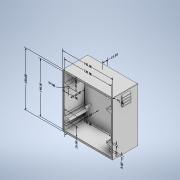
# Autodesk Inventor part: Part_B1
Saved by Autodesk Inventor 2022.6 (Build 266554010, 554A)
## iProperties
Created: 2025-05-15
Part Number: Part_B1
Material: Generic
Document SubType Name: Modeling
Designer: khinm
Density: 1 g/cm^3
Appearance: Default
Author: khinm
Autodesk Inventor part; units mm, degrees
sketch "Sketch1" plane through (0, 0, 0) normal (0, 0, 1) x (1, 0, 0)
  line L0 (-70, 75) -> (70, 75)
  line L1 (70, 75) -> (70, -75)
  line L2 (70, -75) -> (-70, -75)
  line L3 (-70, -75) -> (-70, 75)
  point P0 (0, 0)
  point P1 (-70, 0)
  point P2 (0, 75)
  dimension "d0" = 150
  dimension "d1" = 140
  constraints: 8 end point, 2 midpoint, 2 parallel, 1 horizontal, 1 horizontal alignment, 1 perpendicular, 1 vertical alignment
  measures "d0" distance between parallel lines of L2 L0
  measures "d1" distance between parallel lines of L1 L3
extrude "Extrusion1" add sketch "Sketch1" along normal mid plane 70
sketch "Sketch2" plane through (0, 0, 35) normal (0, 0, 1) x (1, 0, 0)
  line L0 (-65, 70) -> (65, 70)
  line L1 (65, 70) -> (65, -70)
  line L2 (65, -70) -> (-65, -70)
  line L3 (-65, -70) -> (-65, 70)
  point P0 (0, 0)
  point P1 (-65, 0)
  point P2 (0, 70)
  dimension "d4" = 130
  dimension "d5" = 140
  constraints: 8 end point, 2 midpoint, 2 parallel, 1 horizontal, 1 horizontal alignment, 1 perpendicular, 1 vertical alignment
  measures "d4" distance of L0.start L0.end
  measures "d5" distance of L0.end L1.end
extrude "Extrusion2" cut sketch "Sketch2" against normal blind 55
sketch "Sketch4" plane through (0, 0, -20) normal (0, 0, 1) x (1, 0, 0)
  arc A0 (-55, 36) -> (-55, 44) centre (-55, 40) ccw
  arc A1 (-55, -44) -> (-55, -36) centre (-55, -40) ccw
  line L0 (-65, 70) -> (65, 70) projected
  line L1 (65, -70) -> (-65, -70) projected
  line L2 (-65, -70) -> (-65, 70) projected
  line L3 (-55, 44) -> (-65, 44)
  line L4 (-55, 36) -> (-65, 36)
  line L5 (-65, -70) -> (-65, 70) projected
  line L6 (-55, -36) -> (-65, -36)
  line L7 (-55, -44) -> (-65, -44)
  line L8 (-65, 44) -> (-65, 36)
  line L9 (-65, -36) -> (-65, -44)
  point P0 (0, 0)
  point P1 (-60, -36)
  dimension "d11" = 30
  dimension "d12" = 30
  dimension "d13" = 10
  dimension "d14" = 10
  dimension "d15" = 8
  dimension "d16" = 8
  dimension "d100" = 34
  constraints: 12 end point, 4 point on circle, 4 point on line, 3 parallel, 3 perpendicular, 2 centre point, 2 collinear, 2 tangent, 1 midpoint
  measures "d11" distance from line of L0 A0.centre
  measures "d12" distance from line of L1 A1.centre
  measures "d13" distance from line of L2 A0.centre
  measures "d14" distance from line of L2 A1.centre
  measures "d15" diameter of A0
  measures "d16" diameter of A1
  measures "d100" distance from line of L1 point (-60, -36)
extrude "Extrusion3" add sketch "Sketch4" along normal up to surface (55 mm away)
mirror "Mirror1" about plane through (0, 0, 0) normal (1, 0, 0) of "Extrusion3"
sketch "Sketch8" plane through (0, 0, 35) normal (0, 0, 1) x (1, 0, 0)
  line L0 (65, 70) -> (65, 44) projected
  line L1 (65, 44) -> (55, 44) projected
  arc A0 (55, 44) -> (55, 36) centre (55, 40) ccw projected
  line L2 (55, 36) -> (65, 36) projected
  line L3 (65, 36) -> (65, -36) projected
  line L4 (65, -36) -> (55, -36) projected
  arc A1 (55, -36) -> (55, -44) centre (55, -40) ccw projected
  line L5 (55, -44) -> (65, -44) projected
  line L6 (65, -44) -> (65, -70) projected
  line L7 (65, -70) -> (-65, -70) projected
  line L8 (-65, -70) -> (-65, -44) projected
  line L9 (-55, -44) -> (-65, -44) projected
  arc A2 (-55, -44) -> (-55, -36) centre (-55, -40) ccw projected
  line L10 (-65, -36) -> (-55, -36) projected
  line L11 (-65, -36) -> (-65, 36) projected
  line L12 (-55, 36) -> (-65, 36) projected
  arc A3 (-55, 36) -> (-55, 44) centre (-55, 40) ccw projected
  line L13 (-65, 44) -> (-55, 44) projected
  line L14 (-65, 44) -> (-65, 70) projected
  line L15 (-65, 70) -> (65, 70) projected
  line L16 (-70, -75) -> (70, -75) projected
  line L17 (70, -75) -> (70, 75) projected
  line L18 (70, 75) -> (-70, 75) projected
  line L19 (-70, 75) -> (-70, -75) projected
  point P0 (0, 0)
  constraints: 2 coincident
hole "Hole3" at (-55, -40, 35) at (-55, 40, 35) direction (0, 0, -1) diameter 2.013 depth 55
mirror "Mirror3" about plane through (0, 0, 0) normal (1, 0, 0) of "Hole3"
sketch "Sketch9" plane through (0, 0, -20) normal (0, 0, 1) x (1, 0, 0)
  line L0 (-50, 65) -> (50, 65)
  line L1 (50, 65) -> (50, -30)
  line L2 (50, -30) -> (-50, -30)
  line L3 (-50, -30) -> (-50, 65)
  line L4 (-65, 70) -> (65, 70) projected
  circle A0 centre (-47.5, 62.5) radius 2.5
  circle A1 centre (47.5, 62.5) radius 2.5
  circle A2 centre (-47.5, -27.5) radius 2.5
  circle A3 centre (47.5, -27.5) radius 2.5
  point P0 (0, 0)
  point P1 (0, 65)
  dimension "d40" = 100
  dimension "d41" = 95
  dimension "d42" = 5
  dimension "d43" = 2.5
  dimension "d44" = 2.5
  dimension "d45" = 2.5
  dimension "d46" = 2.5
  dimension "d47" = 2.5
  dimension "d48" = 2.5
  dimension "d49" = 2.5
  dimension "d50" = 2.5
  dimension "d51" = 5
  dimension "d52" = 5
  dimension "d53" = 5
  dimension "d54" = 5
  constraints: 8 end point, 4 centre point, 2 parallel, 1 horizontal, 1 midpoint, 1 perpendicular, 1 vertical alignment
  measures "d40" distance of L0.start L0.end
  measures "d41" distance of L0.end L1.end
  measures "d42" distance between parallel lines of L0 L4
  measures "d43" distance from line of L0 A0.centre
  measures "d44" distance from line of L3 A0.centre
  measures "d45" distance from line of L0 A1.centre
  measures "d46" distance from line of L1 A1.centre
  measures "d47" distance from line of L2 A2.centre
  measures "d48" distance from line of L3 A2.centre
  measures "d49" distance from line of L2 A3.centre
  measures "d50" distance from line of L1 A3.centre
  measures "d51" diameter of A0
  measures "d52" diameter of A1
  measures "d53" diameter of A2
  measures "d54" diameter of A3
extrude "Extrusion4" add sketch "Sketch9" along normal blind 15 contours A0 | A1 | A2 | A3
sketch "Sketch10" plane through (-47.5, 62.5, -5) normal (0, 0, 1) x (1, 0, 0)
  circle A0 centre (0, 0) radius 2.5 projected
  point P0 (47.5, -62.5)
  constraints: 1 coincident
sketch "Sketch11" plane through (-47.5, -27.5, -5) normal (0, 0, 1) x (1, 0, 0)
  circle A0 centre (0, 0) radius 2.5 projected
  point P0 (47.5, 27.5)
  constraints: 1 coincident
sketch "Sketch12" plane through (47.5, 62.5, -5) normal (0, 0, 1) x (1, 0, 0)
  circle A0 centre (0, 0) radius 2.5 projected
  point P0 (-47.5, -62.5)
  constraints: 1 coincident
sketch "Sketch13" plane through (47.5, -27.5, -5) normal (0, 0, 1) x (1, 0, 0)
  circle A0 centre (0, 0) radius 2.5 projected
  point P0 (-47.5, 27.5)
  constraints: 1 coincident
hole "Hole4" at (-47.5, 62.5, -5) direction (0, 0, -1) diameter 2.013 depth 15
hole "Hole5" at (-47.5, -27.5, -5) direction (0, 0, -1) diameter 2.013 depth 15
hole "Hole6" at (47.5, -27.5, -5) direction (0, 0, -1) diameter 2.013 depth 15
hole "Hole7" at (47.5, 62.5, -5) direction (0, 0, -1) diameter 2.013 depth 15
ref_plane "Work Plane2" through (0, 0, 0) normal (1, 0, 0) x (0, 1, 0)
sketch "Sketch15" plane through (0, 0, 0) normal (1, 0, 0) x (0, 1, 0)
  line L0 (75, 35) -> (-75, 35) projected
  line L1 (73.5, 35) -> (71.5, 35)
  line L2 (71.5, 35) -> (71.5, 28)
  line L3 (71.5, 28) -> (73.5, 28)
  line L4 (73.5, 28) -> (73.5, 35)
  line L5 (75, -35) -> (75, 35) projected
  point P0 (0, 0)
  point P1 (73.5, 31.5)
  point P2 (72.5, 35)
  dimension "d105" = 2
  dimension "d106" = 1.5
  dimension "d107" = 0
  dimension "d108" = 7
  constraints: 8 end point, 2 midpoint, 2 parallel, 1 horizontal, 1 perpendicular
  measures "d105" distance between parallel lines of L2 L4
  measures "d106" distance from line of L5 point (73.5, 31.5)
  measures "d107" distance from line of L0 point (72.5, 35)
  measures "d108" distance of L2.end L1.end
sketch3d "3D Sketch1"
  line L0 (70, 75, 35) -> (70, -75, 35)
  line L1 (70, -75, 35) -> (-70, -75, 35)
  line L2 (-70, -75, 35) -> (-70, 75, 35)
  line L3 (-70, 75, 35) -> (70, 75, 35)
sweep "Sweep1" cut profiles "Sketch15" path "3D Sketch1"
sketch "Sketch16" plane through (0, 0, -20) normal (0, 0, 1) x (1, 0, 0)
  line L0 (65, 36) -> (65, -36) projected
  circle A0 centre (-47.5, 62.5) radius 2.5 projected
  circle A1 centre (47.5, -27.5) radius 2.5 projected
  circle A2 centre (47.5, 62.5) radius 2.5 projected
  circle A3 centre (-47.5, -27.5) radius 2.5 projected
  line L1 (65, -44) -> (55, -44) projected
  arc A4 (55, -36) -> (55, -44) centre (55, -40) ccw projected
  line L2 (55, -36) -> (65, -36) projected
  line L3 (65, 36) -> (65, -36) projected
  line L4 (65, 36) -> (55, 36) projected
  arc A5 (55, 44) -> (55, 36) centre (55, 40) ccw projected
  line L5 (55, 44) -> (65, 44) projected
  line L6 (65, 70) -> (65, 44) projected
  line L7 (-65, 70) -> (65, 70) projected
  line L8 (-65, 44) -> (-65, 70) projected
  line L9 (-65, 44) -> (-55, 44) projected
  arc A6 (-55, 36) -> (-55, 44) centre (-55, 40) ccw projected
  line L10 (-55, 36) -> (-65, 36) projected
  line L11 (-65, -36) -> (-65, 36) projected
  line L12 (-65, -36) -> (-55, -36) projected
  arc A7 (-55, -44) -> (-55, -36) centre (-55, -40) ccw projected
  line L13 (-55, -44) -> (-65, -44) projected
  line L14 (-65, -70) -> (-65, -44) projected
  line L15 (65, -70) -> (-65, -70) projected
  line L16 (65, -44) -> (65, -70) projected
  line L17 (60, -31) -> (65, -31)
  line L18 (65, -31) -> (65, -32.5)
  line L19 (65, -32.5) -> (60, -32.5)
  line L20 (60, -32.5) -> (60, -31)
  line L21 (60, -49.5) -> (65, -49.5)
  line L22 (65, -49.5) -> (65, -51)
  line L23 (65, -51) -> (60, -51)
  line L24 (60, -51) -> (60, -49.5)
  line L25 (60, -56) -> (65, -56)
  line L26 (65, -56) -> (65, -57.5)
  line L27 (65, -57.5) -> (60, -57.5)
  line L28 (60, -57.5) -> (60, -56)
  point P0 (0, 0)
  point P1 (65, -31.75)
  point P2 (62.5, -49.5)
  point P3 (65, -50.25)
  point P4 (62.5, -51)
  point P5 (62.5, -56)
  point P6 (65, -56.75)
  dimension "d111" = 3.5
  dimension "d112" = 0
  dimension "d113" = 5
  dimension "d114" = 1.5
  dimension "d115" = 5.5
  dimension "d116" = 5
  constraints: 24 end point, 6 midpoint, 6 parallel, 4 equal length, 3 horizontal, 3 perpendicular, 2 vertical alignment
  measures "d111" distance between parallel lines of L19 L2
  measures "d112" distance from line of L3 point (65, -31.75)
  measures "d113" distance of L18.end L19.end
  measures "d114" distance between parallel lines of L19 L17
  measures "d115" distance from line of point (62.5, -49.5) L1
  measures "d116" distance of point (62.5, -51) point (62.5, -56)
extrude "Extrusion6" add sketch "Sketch16" along normal up to surface (55 mm away) contours L0 L19 L20 L17 | L16 L23 L24 L21 | L16 L27 L28 L25
mirror "Mirror4" about plane through (0, 0, 0) normal (1, 0, 0) of "Extrusion6"
fillet "Fillet2" radius 1 4 edges at (70, 75, 0) (70, -75, 0) (-70, 75, 0) (-70, -75, 0)
sketch "Sketch17" plane through (0, 0, -20) normal (0, 0, 1) x (1, 0, 0)
  circle A0 centre (0, 55) radius 4
  circle A1 centre (0, 14) radius 4
  line L0 (-65, 70) -> (65, 70) projected
  point P0 (0, 0)
  dimension "d121" = 15
  dimension "d122" = 56
  dimension "d123" = 8
  dimension "d124" = 8
  constraints: 2 centre point, 2 vertical alignment, 1 equal radius
  measures "d121" distance from line of A0.centre L0
  measures "d122" distance from line of A1.centre L0
  measures "d123" diameter of A0
  measures "d124" diameter of A1
extrude "Extrusion7" cut sketch "Sketch17" against normal up to surface (15 mm away)
sketch "Sketch18" plane through (0, 0, -35) normal (0, 0, -1) x (-1, 0, 0)
  line L0 (-3.5, 40) -> (3.5, 40)
  point P0 (0, 0)
  point P1 (0, 40)
  dimension "d127" = 7
  dimension "d128" = 40
  constraints: 2 coincident, 2 end point, 1 horizontal, 1 midpoint, 1 vertical alignment
  measures "d127" distance of L0.start L0.end
  measures "d128" distance of point (0, 40) point (0, 0)
hole "Hole8" at (3.5, 40, -35) at (-3.5, 40, -35) direction (0, 0, 1) diameter 2.013 depth 10
pattern_linear "Rectangular Pattern1" count 2 spacing 100 along (0, -1, 0) of "Hole8"
ref_plane "Work Plane3" through (0, 0, 0) normal (0, 0, 1) x (1, 0, 0)
sketch "Sketch19" plane through (0, 0, 0) normal (0, 0, 1) x (1, 0, 0)
  line L0 (65, 68) -> (70, 68)
  line L1 (70, 68) -> (70, 66)
  line L2 (70, 66) -> (65, 66)
  line L3 (65, 66) -> (65, 68)
  line L4 (65, 61) -> (70, 61)
  line L5 (70, 61) -> (70, 59)
  line L6 (70, 59) -> (65, 59)
  line L7 (65, 59) -> (65, 61)
  line L8 (65, 54) -> (70, 54)
  line L9 (70, 54) -> (70, 52)
  line L10 (70, 52) -> (65, 52)
  line L11 (65, 52) -> (65, 54)
  line L12 (-65, 70) -> (65, 70) projected
  line L13 (70, 74) -> (70, -74) projected
  line L14 (65, 70) -> (65, 44) projected
  line L15 (65, 47) -> (70, 47)
  line L16 (70, 47) -> (70, 45)
  line L17 (70, 45) -> (65, 45)
  line L18 (65, 45) -> (65, 47)
  point P0 (0, 0)
  point P1 (67.5, 66)
  point P2 (67.5, 68)
  point P3 (70, 67)
  point P4 (65, 67)
  point P5 (65, 53)
  point P6 (65, 46)
  point P7 (70, 53)
  point P8 (70, 46)
  point P9 (70, 45)
  point P10 (70, 47)
  dimension "d143" = 2
  dimension "d144" = 5
  dimension "d145" = 5
  dimension "d146" = 2
  dimension "d147" = 0
  dimension "d148" = 0
  dimension "d149" = 5
  constraints: 32 end point, 8 midpoint, 8 parallel, 4 horizontal, 4 perpendicular, 4 point on line, 3 collinear, 2 vertical alignment
  measures "d143" distance of point (67.5, 66) point (67.5, 68)
  measures "d144" distance of L4.end L1.end
  measures "d145" distance of L8.end L5.end
  measures "d146" distance from line of L12 point (67.5, 68)
  measures "d147" distance from line of L13 point (70, 67)
  measures "d148" distance from line of L14 point (65, 67)
  measures "d149" distance of L15.end L9.end
extrude "Extrusion8" cut sketch "Sketch19" along normal mid plane 20 contours L0 L1 L2 L3 | L4 L5 L6 L7 | L8 L9 L10 L11 | L15 L13 L17 L14
sketch "Sketch20" plane through (0, 0, 0) normal (0, 0, 1) x (1, 0, 0)
  line L0 (65, 68) -> (70, 68) projected
  line L1 (70, 68) -> (70, 68)
  line L2 (72, 66) -> (72, 64)
  line L3 (72, 64) -> (73.5, 64)
  line L4 (73.5, 64) -> (73.5, 66)
  line L5 (70, 69.5) -> (70, 69.5)
  line L6 (70, 69.5) -> (70, 68)
  line L7 (70, 74) -> (70, -74) projected
  arc A0 (72, 66) -> (70, 68) centre (70, 66) ccw
  arc A1 (73.5, 66) -> (70, 69.5) centre (70, 66) ccw
  line L8 (65, 61) -> (70, 61) projected
  line L9 (70, 61) -> (70, 61)
  line L10 (72, 59) -> (72, 57)
  line L11 (72, 57) -> (73.5, 57)
  line L12 (73.5, 57) -> (73.5, 59)
  line L13 (70, 62.5) -> (70, 62.5)
  line L14 (70, 62.5) -> (70, 61)
  line L15 (65, 54) -> (70, 54) projected
  line L16 (70, 54) -> (70, 54)
  line L17 (72, 52) -> (72, 50)
  line L18 (72, 50) -> (73.5, 50)
  line L19 (73.5, 50) -> (73.5, 52)
  line L20 (70, 55.5) -> (70, 55.5)
  line L21 (70, 55.5) -> (70, 54)
  line L22 (70, 47) -> (70, 47)
  line L23 (72, 45) -> (72, 43)
  line L24 (72, 43) -> (73.5, 43)
  line L25 (73.5, 43) -> (73.5, 45)
  line L26 (70, 48.5) -> (70, 48.5)
  line L27 (70, 47) -> (70, 48.5)
  line L28 (65, 47) -> (70, 47) projected
  arc A2 (73.5, 59) -> (70, 62.5) centre (70, 59) ccw
  arc A3 (73.5, 52) -> (70, 55.5) centre (70, 52) ccw
  arc A4 (73.5, 45) -> (70, 48.5) centre (70, 45) ccw
  arc A5 (72, 59) -> (70, 61) centre (70, 59) ccw
  arc A6 (72, 52) -> (70, 54) centre (70, 52) ccw
  arc A7 (72, 45) -> (70, 47) centre (70, 45) ccw
  point P0 (0, 0)
  point P1 (70, 68)
  point P2 (72.75, 64)
  point P3 (72.75, 57)
  point P4 (72, 47)
  point P5 (73.5, 48.5)
  point P6 (71, 47)
  point P7 (72.75, 50)
  point P8 (72.75, 43)
  point P9 (67.5, 47)
  point P10 (70, 54)
  point P11 (67.5, 54)
  point P12 (67.5, 61)
  point P13 (67.5, 68)
  dimension "d158" = 1.5
  dimension "d159" = 1.5
  dimension "d160" = 2
  dimension "d161" = 2
  dimension "d162" = 3.5
  dimension "d163" = 4
  dimension "d164" = 2
  dimension "d165" = 4
  dimension "d166" = 2
  dimension "d168" = 1.5
  dimension "d169" = 4
  dimension "d170" = 4
  dimension "d171" = 3.5
  dimension "d172" = 2
  constraints: 48 end point, 16 point on circle, 16 tangent, 13 perpendicular, 11 midpoint, 9 point on line, 8 centre point, 5 horizontal, 4 equal length, 4 equal radius, 4 horizontal alignment, 4 vertical, 5 other
  measures "d158" distance of L2.end L3.end
  measures "d159" distance from line of point (70, 68) L5
  measures "d161" radius of A0
  measures "d162" radius of A1
  measures "d163" vertical distance of point (72.75, 64) L0.end
  measures "d164" length of L10
  measures "d165" vertical distance of point (72.75, 57) L8.end
  measures "d166" length of L17
  measures "d168" distance from line of point (71, 47) L26
  measures "d169" distance from line of point (72.75, 50) L16
  measures "d170" distance from line of point (72.75, 43) L22
  measures "d171" radius of A2
  measures "d172" radius of A5
extrude "Extrusion9" add sketch "Sketch20" along normal mid plane 20
ref_plane "Work Plane4" through (0, 0, -10) normal (0, 0, 1) x (1, 0, 0)
sketch "Sketch21" plane through (0, 0, -10) normal (0, 0, 1) x (1, 0, 0)
  line L0 (70, -74) -> (70, 74) projected
  arc A0 (73.5, 66) -> (70, 69.5) centre (70, 66) ccw projected
  line L1 (70, 69.5) -> (70, 69.5)
  line L2 (72, 64) -> (73.5, 64) projected
  line L3 (73.5, 66) -> (73.5, 64)
  line L4 (73.5, 64) -> (70, 64)
  line L5 (70, 64) -> (70, 69.5)
  arc A1 (73.5, 66) -> (70, 69.5) centre (70, 66) ccw
  arc A2 (73.5, 59) -> (70, 62.5) centre (70, 59) ccw projected
  line L6 (70, 62.5) -> (70, 62.5)
  line L7 (73.5, 57) -> (73.5, 59) projected
  line L8 (73.5, 59) -> (73.5, 57)
  line L9 (73.5, 57) -> (70, 57)
  line L10 (70, 57) -> (70, 62.5)
  arc A3 (73.5, 52) -> (70, 55.5) centre (70, 52) ccw projected
  line L11 (70, 55.5) -> (70, 55.5)
  line L12 (73.5, 50) -> (73.5, 52) projected
  line L13 (73.5, 52) -> (73.5, 50)
  line L14 (73.5, 50) -> (70, 50)
  line L15 (70, 50) -> (70, 55.5)
  arc A4 (73.5, 45) -> (70, 48.5) centre (70, 45) ccw projected
  line L16 (70, 48.5) -> (70, 48.5)
  line L17 (72, 43) -> (73.5, 43) projected
  line L18 (73.5, 45) -> (73.5, 43)
  line L19 (73.5, 43) -> (70, 43)
  line L20 (70, 43) -> (70, 48.5)
  arc A5 (73.5, 59) -> (70, 62.5) centre (70, 59) ccw
  arc A6 (73.5, 52) -> (70, 55.5) centre (70, 52) ccw
  arc A7 (73.5, 45) -> (70, 48.5) centre (70, 45) ccw
  point P0 (0, 0)
  point P1 (73.5, 55.5)
  point P2 (73.5, 48.5)
  point P3 (73.5, 66)
  dimension "d176" = 3.5
  dimension "d177" = 3.5
  constraints: 32 end point, 11 tangent, 8 point on circle, 6 perpendicular, 6 point on line, 5 vertical, 4 centre point, 4 horizontal, 2 equal radius, 1 collinear, 5 other
  measures "d176" radius of A1
  measures "d177" radius of A5
extrude "Extrusion10" add sketch "Sketch21" against normal blind 2
mirror "Mirror5" about plane through (0, 0, 0) normal (0, 0, 1) of "Extrusion10"
mirror "Mirror6" about plane through (0, 0, 0) normal (1, 0, 0) of "Extrusion9", "Extrusion10", "Mirror5", "Extrusion8"
fillet "Fillet3" radius 1 8 edges at (69.7071, 74.7071, -35) (70, 0, -35) (69.7071, -74.7071, -35) (0, -75, -35) (-69.7071, -74.7071, -35) (-70, 0, -35) (-69.7071, 74.7071, -35) (0, 75, -35)
body "Solid1"
